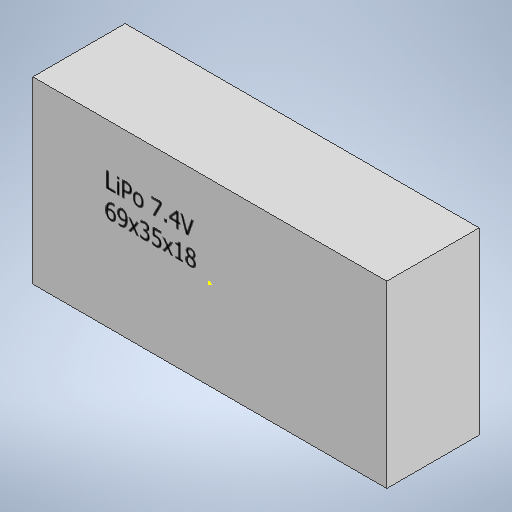
# Autodesk Inventor part: LiPo-7.4V-69x35x18
Saved by Autodesk Inventor 2025.3 (Build 293356030, 356C)
## iProperties
Created: 2025-08-30
Part Number: LiPo-7.4V-69x35x18
Material: 一般
Document SubType Name: Modeling
Designer: daisuke
Density: 1 g/cm^3
Appearance: 既定
Author: daisuke
Autodesk Inventor part; units mm, degrees
ref_plane "YZ Plane" through (0, 0, 0) normal (1, 0, 0) x (0, 1, 0)
ref_plane "XZ Plane" through (0, 0, 0) normal (0, 1, 0) x (-1, 0, 0)
ref_plane "XY Plane" through (0, 0, 0) normal (0, 0, 1) x (1, 0, 0)
sketch "スケッチ1" plane through (0, 0, 0) normal (0, 0, 1) x (1, 0, 0)
  line L0 (-34.5, 17.5) -> (34.5, 17.5)
  line L1 (34.5, 17.5) -> (34.5, -17.5)
  line L2 (34.5, -17.5) -> (-34.5, -17.5)
  line L3 (-34.5, -17.5) -> (-34.5, 17.5)
  point P0 (0, 0)
  point P1 (0, 17.5)
  point P2 (-34.5, 0)
  dimension "d0" = 69
  dimension "d1" = 35
  constraints: 8 end point, 2 midpoint, 2 parallel, 1 horizontal, 1 horizontal alignment, 1 perpendicular, 1 vertical alignment
  measures "d0" distance of L1.end L2.end
  measures "d1" distance of L0.end L1.end
extrude "押し出し1" add sketch "スケッチ1" along normal blind 18
sketch "スケッチ2" plane through (0, 0, 18) normal (0, 0, 1) x (1, 0, 0)
  line L0 (-20.4486, 8.918) -> (24.838, 8.918) construction
  line L1 (24.838, 8.918) -> (24.838, -6.4098) construction
  line L2 (24.838, -6.4098) -> (-20.4486, -6.4098) construction
  line L3 (-20.4486, -6.4098) -> (-20.4486, 8.918) construction
  point P0 (0, 0)
  constraints: 2 other
